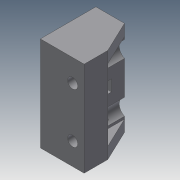
# Autodesk Inventor part: FLUGGER FRT UPSTOP FLAP 
Saved by Autodesk Inventor 2020.3 (Build 243373000, 373)
## iProperties
RuleStatus: InUse
AfterDocSave0: file://Part Number Cleaner
Created: 2019-11-18
Material: Generic
Vendor: HHMI: JRC - ID&F
Document SubType Name: Modeling
Designer: arnoldj
Density: 1 g/cm^3
Appearance: Default
DESIGN DEPARTMENT: HHMI: JRC - ID&F
ALTERED ITEM PART NUMBER: N/A
ALTERED ITEM VENDOR: N/A
ALTERED ITEM DESCRIPTION: N/A
Author: arnoldj
Revision Number: 0
Autodesk Inventor part; units mm, degrees
ref_plane "YZ Plane" through (0, 0, 0) normal (1, 0, 0) x (0, 1, 0)
ref_plane "XZ Plane" through (0, 0, 0) normal (0, 1, 0) x (-1, 0, 0)
ref_plane "XY Plane" through (0, 0, 0) normal (0, 0, 1) x (1, 0, 0)
sketch "Sketch1" plane through (0, 0, 0) normal (0, 1, 0) x (-1, 0, 0)
  line L0 (0, -29.5656) -> (0, 4.9276) projected
  line L1 (-23.3172, 0) -> (3.8862, 0) projected
  line L2 (0, 0) -> (-19.431, 0)
  line L3 (-19.431, 0) -> (-19.431, -10.4775)
  line L4 (-19.431, -10.4775) -> (0, -10.4775)
  line L5 (0, -10.4775) -> (0, 0)
  line L6 (0, -10.4775) -> (-12.7, -10.4775)
  line L7 (-12.7, -10.4775) -> (-12.7, -24.638)
  line L8 (0, -24.638) -> (0, -10.4775)
  line L9 (0, -24.638) -> (-12.7, -24.638)
  dimension "d10" = 10.4775
  dimension "d36" = 24.638
  dimension "d37" = 12.7
  dimension "d38" = 19.431
  constraints: 16 end point, 3 parallel, 3 perpendicular, 2 horizontal, 2 point on line
  measures "d10" distance of L2.end L3.end
  measures "d36" distance between parallel lines of L9 L1
  measures "d37" distance of L8.start L7.end
  measures "d38" distance between parallel lines of L0 L3
extrude "Extrusion3" add sketch "Sketch1" along normal mid plane 41.91
sketch "Sketch2" plane through (19.431, 20.955, -24.638) normal (0, 0, -1) x (-1, 0, 0)
  line L0 (6.731, -41.91) -> (6.731, 0) projected
  line L1 (0, 0) -> (6.731, 0) projected
  line L2 (0, -41.91) -> (0, 0) projected
  line L3 (6.731, -41.91) -> (0, -41.91) projected
  line L4 (-3.8862, -20.955) -> (23.3172, -20.955) projected
  line L5 (19.431, -41.91) -> (19.431, 0) projected
  point P0 (19.431, -20.955)
  point P1 (5.08, -9.8425)
  point P2 (5.08, -32.0675)
  dimension "d73" = 22.225
  dimension "d74" = 11.1125
  dimension "d75" = 14.351
  measures "d73" distance of point (5.08, -32.068) point (5.08, -9.842)
  measures "d74" distance from line of point (5.08, -9.842) L4
  measures "d75" distance from line of point (5.08, -9.842) L5
hole "Hole1" at (14.351, 11.1125, -24.638) at (14.351, -11.1125, -24.638) direction (0, 0, 1) diameter 4.4958 end through all counterbore diameter 8.001 counterbore depth 14.1605 clearance for "Socket Head Cap Screw" size "M4" standard "Ansi Metric M Profile"
sketch "Sketch3" plane through (0, -20.955, 0) normal (0, 1, 0) x (-1, 0, 0)
  line L0 (-12.7, -24.638) -> (-12.7, -10.4775) projected
  line L1 (-12.7, -10.4775) -> (-19.431, -10.4775) projected
  line L2 (-19.431, -10.4775) -> (-12.7, -24.638)
  line L3 (-12.7, -24.638) -> (-12.7, -10.4775)
  line L4 (-19.431, -10.4775) -> (-12.7, -10.4775)
  point P0 (0, 0)
  constraints: 6 end point, 1 horizontal, 1 vertical
extrude "Extrusion4" add sketch "Sketch3" along normal blind 5.08
sketch "Sketch4" plane through (12.7, 20.955, -24.638) normal (0, 0, -1) x (-1, 0, 0)
  line L0 (12.7, -50.292) -> (12.7, 8.382) projected
  line L1 (-10.6172, -20.955) -> (16.5862, -20.955) projected
  line L2 (0, -6.1986) -> (0, 0) projected
  point P0 (12.7, -20.955)
  point P1 (6.35, -9.525)
  point P2 (6.35, -32.385)
  point P3 (6.35, -20.955)
  point P4 (0, -36.83)
  dimension "d39" = 11.43
  dimension "d40" = 11.43
  dimension "d41" = 6.35
  dimension "d63" = 12.7
  constraints: 2 vertical alignment, 1 point on line
  measures "d39" distance from line of point (6.35, -9.525) L1
  measures "d40" distance from line of L1 point (6.35, -32.385)
  measures "d41" distance from line of point (6.35, -9.525) L0
  measures "d63" distance between parallel lines of L0 L2
hole "Hole2" at (6.35, 11.43, -24.638) at (6.35, -11.43, -24.638) at (6.35, 0, -24.638) direction (0, 0, 1) diameter 2.54 depth 10.922 tip angle 118 clearance for "Flat Head Machine Screw (100)" size "#2" standard "Ansi Unified Screw Threads"
sketch "Sketch5" plane through (12.7, 20.955, -10.4775) normal (1, 0, 0) x (0, 0, -1)
  line L0 (-15.4051, -20.955) -> (19.0881, -20.955) projected
  line L1 (-10.4775, -50.292) -> (-10.4775, 8.382) projected
  line L2 (6.5405, -12.0396) -> (8.3693, -12.0396)
  line L3 (8.3693, -12.0396) -> (8.3693, -7.0104)
  line L4 (8.3693, -7.0104) -> (6.5405, -7.0104)
  line L5 (6.5405, -7.0104) -> (6.5405, -12.0396)
  line L6 (6.5405, -12.0396) -> (8.3693, -7.0104) construction
  line L7 (8.3693, -12.0396) -> (6.5405, -7.0104) construction
  line L8 (6.5405, -23.4696) -> (8.3693, -23.4696)
  line L9 (8.3693, -23.4696) -> (8.3693, -18.4404)
  line L10 (8.3693, -18.4404) -> (6.5405, -18.4404)
  line L11 (6.5405, -18.4404) -> (6.5405, -23.4696)
  line L12 (6.5405, -23.4696) -> (8.3693, -18.4404) construction
  line L13 (8.3693, -23.4696) -> (6.5405, -18.4404) construction
  line L14 (6.5405, -34.8996) -> (8.3693, -34.8996)
  line L15 (8.3693, -34.8996) -> (8.3693, -29.8704)
  line L16 (8.3693, -29.8704) -> (6.5405, -29.8704)
  line L17 (6.5405, -29.8704) -> (6.5405, -34.8996)
  line L18 (6.5405, -34.8996) -> (8.3693, -29.8704) construction
  line L19 (8.3693, -34.8996) -> (6.5405, -29.8704) construction
  line L20 (14.1605, -6.1986) -> (14.1605, 0) projected
  point P0 (-10.4775, -20.955)
  point P1 (7.4549, -9.525)
  point P2 (7.4549, -20.955)
  point P3 (7.4549, -32.385)
  point P4 (14.1605, -36.83)
  point P5 (7.4549, -9.525)
  point P6 (7.4549, -32.385)
  dimension "d49" = 5.0292
  dimension "d50" = 1.8288
  dimension "d51" = 11.43
  dimension "d58" = 7.62
  dimension "d59" = 11.43
  constraints: 36 end point, 8 midpoint, 6 parallel, 4 equal length, 3 horizontal, 3 perpendicular, 2 point on line, 1 vertical alignment
  measures "d49" distance of L2.end L3.end
  measures "d50" distance of L3.end L4.end
  measures "d51" distance from line of L0 point (7.455, -9.525)
  measures "d58" distance between parallel lines of L20 L5
  measures "d59" distance from line of L0 point (7.455, -32.385)
extrude "Extrusion5" cut sketch "Sketch5" along normal blind 10.16 and the other way blind 9.144
sketch "Sketch6" plane through (0, 20.955, 0) normal (0, 1, 0) x (1, 0, 0)
  line L0 (12.7, 10.4775) -> (12.7, 24.638) projected
  line L1 (19.431, 10.4775) -> (12.7, 10.4775) projected
  line L2 (19.431, 10.4775) -> (12.7, 24.638) projected
  point P0 (0, 0)
extrude "Extrusion6" add sketch "Sketch6" against normal blind 5.08
sketch "Sketch7" plane through (0, 20.955, 0) normal (0, 1, 0) x (1, 0, 0)
  line L0 (0, 0) -> (19.431, 0) projected
  line L1 (19.431, 0) -> (19.431, 10.4775) projected
  line L2 (7.7406, 0) -> (19.5357, -3.1605)
  line L3 (19.5357, -3.1605) -> (19.431, 0)
  line L4 (7.7406, 0) -> (19.431, 0)
  dimension "d64" = 11.684
  dimension "d65" = 15
  constraints: 6 end point, 1 horizontal, 1 point on line
  measures "d64" distance from line of L2.start L3
  measures "d65" angle of L0 L2
extrude "Extrusion7" [suppressed]
sketch "Sketch8" plane through (19.431, -20.955, 0) normal (1, 0, 0) x (0, 0, -1)
  line L0 (10.4775, 0) -> (10.4775, 5.08) projected
  line L1 (10.4775, 5.08) -> (10.4775, 36.83) projected
  line L2 (10.4775, 36.83) -> (10.4775, 41.91) projected
  line L3 (0, 41.91) -> (10.4775, 41.91) projected
  line L4 (0, 0) -> (0, 41.91) projected
  line L5 (10.4775, 0) -> (0, 0) projected
  line L6 (10.4775, 41.91) -> (-3.81, 41.91)
  line L7 (-3.81, 41.91) -> (-3.81, 0)
  line L8 (-3.81, 0) -> (10.4775, 0)
  line L9 (10.4775, 0) -> (10.4775, 41.91)
  point P0 (0, 20.955)
  dimension "d68" = 0
  dimension "d69" = 3.81
  constraints: 8 end point, 2 parallel, 1 horizontal, 1 perpendicular
  measures "d68" distance between parallel lines of L5 L8
  measures "d69" distance between parallel lines of L4 L7
extrude "Extrusion8" [suppressed]
fillet "Fillet2" [suppressed]
equation "\"d74\" = 0.5 * d73"
equation "\"d23\" = d36 - d10"
equation "\"d40\" = d39"
equation "\"d41\" = 0.5 * d63"
body "Solid2"
